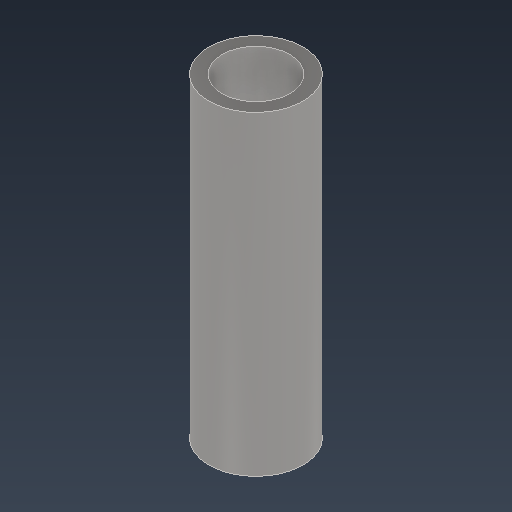
# Autodesk Inventor part: SP5V1 Camisa Freno
Saved by Autodesk Inventor 2021.2 (Build 252289000, 289)
## iProperties
Created: 2026-06-23
Part Number: SP5V1 Camisa Freno
Material: Stainless Steel
Document SubType Name: Modeling
Designer: nelso
Density: 8.08 g/cm^3
Appearance: Semi-Polished
Mass: 58.6372 g
Surface Area: 60.4757 cm^2
Volume: 7.25708 cm^3
Author: nelso
Autodesk Inventor part; units mm, degrees
ref_plane "YZ Plane" through (0, 0, 0) normal (1, 0, 0) x (0, 1, 0)
ref_plane "XZ Plane" through (0, 0, 0) normal (0, 1, 0) x (-1, 0, 0)
ref_plane "XY Plane" through (0, 0, 0) normal (0, 0, 1) x (1, 0, 0)
sketch "Sketch1" plane through (0, 0, 0) normal (0, 1, 0) x (-1, 0, 0)
  circle A0 centre (0, 0) radius 6.45
  circle A1 centre (0, 0) radius 8.95
  dimension "d0" = 12.9
  dimension "d1" = 17.9
  constraints: 2 centre point, 2 coincident
  measures "d0" diameter of A0
  measures "d1" diameter of A1
extrude "Extrusion1" add sketch "Sketch1" along normal mid plane 60
body "Solid1"
